ikea-stolmen-hook-three-pieces (Autodesk Fusion 360 design; units mm, degrees)
Autodesk Fusion 360 part; units mm, degrees
note: some values were not read from the file. Set by a fixed rule: which sketch regions a step uses.
sketch "Sketch1" plane through (0, 0, 0) normal (0, 1, 0) x (1, 0, 0) in component "Component"
  circle A0 centre (0, 0) radius 23.5
  circle A1 centre (0, 0) radius 27.5
  line L0 (-5, 35.5) -> (-9, 35.5)
  line L1 (-9, 35.5) -> (-9, 23.5)
  line L2 (-9, 23.5) -> (-5, 23.5)
  line L3 (-5, 23.5) -> (-5, 35.5)
  line L4 (0, 5) -> (0, -5)
  line L5 (-5, 0) -> (5, 0)
  line L6 (9, 35.5) -> (9, 23.5)
  line L7 (5, 23.5) -> (5, 35.5)
  line L8 (9, 23.5) -> (5, 23.5)
  line L9 (5, 35.5) -> (9, 35.5)
  line L10 (-9, -35.5) -> (-9, -23.5)
  line L11 (-5, -23.5) -> (-5, -35.5)
  line L12 (5, -23.5) -> (5, -35.5)
  line L13 (9, -35.5) -> (9, -23.5)
  line L14 (5, -35.5) -> (9, -35.5)
  line L15 (9, -23.5) -> (5, -23.5)
  line L16 (-9, -23.5) -> (-5, -23.5)
  line L17 (-5, -35.5) -> (-9, -35.5)
  line L18 (-5, 23.5) -> (-5, -23.5)
  line L19 (5, -23.5) -> (5, 23.5)
  dimension "d2" = 47
  dimension "d4" = 55
  dimension "d7" = 4
  dimension "d54" = 12
  measures "d2" diameter of A0
  measures "d4" diameter of A1
  measures "d7" distance of L0.start L0.end
  measures "d54" distance of L0.end L1.end
extrude "Extrude1" add sketch "Sketch1" along normal blind 10 contours A0 A1 L6 L8 L13 L15 L19 | A1 L6 L7 L8 | A1 L12 L13 L15 | A1 L6 L7 L9 | A1 L12 L13 L14 makes body 1 in component "Component"
sketch "Sketch6" plane through (9, 0, 0) normal (1, 0, 0) x (0, 0, -1)
  line L0 (-35.5, 0) -> (-25.9856, 0)
  line L1 (-25.9856, 0) -> (-25.9856, 10)
  line L2 (-25.9856, 10) -> (-35.5, 10)
  line L3 (-35.5, 10) -> (-35.5, 0)
  line L4 (-35.5, 5) -> (-25.9856, 5)
  circle A0 centre (-30.7428, 5) radius 1.6
  line L5 (-30.7428, 8.2) -> (-33.5141, 6.6)
  line L6 (-33.5141, 6.6) -> (-33.5141, 3.4)
  line L7 (-33.5141, 3.4) -> (-30.7428, 1.8)
  line L8 (-30.7428, 1.8) -> (-27.9715, 3.4)
  line L9 (-27.9715, 3.4) -> (-27.9715, 6.6)
  line L10 (-27.9715, 6.6) -> (-30.7428, 8.2)
  line L11 (-30.7428, 7.4) -> (-31.9354, 6.0667)
  line L12 (-30.7428, 7.4) -> (-29.5502, 6.0667)
  point P0 (-30.7428, 5)
  dimension "d72" = 3.2
  dimension "d78" = 2.4
  measures "d72" diameter of A0
  measures "d78" distance of P0 L11.start
sketch "Sketch7" plane through (9, 0, 0) normal (1, 0, 0) x (0, 0, -1)
  line L0 (25.9856, 0) -> (35.5, 0)
  line L1 (35.5, 0) -> (35.5, 10)
  line L2 (35.5, 10) -> (25.9856, 10)
  line L3 (25.9856, 10) -> (25.9856, 0)
  line L4 (25.9856, 5) -> (35.5, 5)
  circle A0 centre (30.7428, 5) radius 1.6
  line L5 (30.7428, 5) -> (30.7428, 7.4)
  line L6 (30.7428, 7.4) -> (29.5502, 6.0667)
  line L7 (30.7428, 7.4) -> (31.9354, 6.0667)
  dimension "d73" = 3.2
  dimension "d79" = 2.4
  measures "d73" diameter of A0
  measures "d79" distance of A0.centre L5.end
extrude "Extrude5" cut sketch "Sketch6" against normal up to surface (4 mm away) contours L4 A0 | L4 A0 | A0 L11 L12 bodies 1 in component "Component"
extrude "Extrude6" cut sketch "Sketch7" against normal up to surface (4 mm away) contours L4 A0 L5 | L4 A0 | L4 A0 L5 | A0 L5 L6 | A0 L5 L7 bodies 1 in component "Component"
extrude "Extrude7" cut sketch "Sketch6" against normal blind 1.5 contours L4 A0 L5 L6 L9 L10 L11 L12 | L4 A0 L6 L7 L8 L9 | A0 L11 L12 bodies 1 in component "Component"
sketch "Sketch5" plane through (0, 0, 0) normal (0, 1, 0) x (1, 0, 0)
  circle A0 centre (-14.9966, 15) radius 5
  line L0 (-19.9966, 15) -> (-19.9966, 0)
  line L1 (-9.9966, 15) -> (-9.9966, 0)
  circle A1 centre (-14.9966, 15) radius 1.6
  line L2 (-14.9966, 2) -> (-6.4966, 2)
  line L3 (-6.4966, 2) -> (-6.4966, -2)
  line L4 (-6.4966, -2) -> (-14.9966, -2)
  line L5 (-14.9966, -2) -> (-14.9966, 2)
  line L6 (-19.9966, 0) -> (-9.9966, 0)
  arc A2 (-49.9966, 0) -> (-19.9966, 0) centre (-34.9966, 0) ccw
  line L7 (-34.9966, 0) -> (-49.9966, 0) construction
  line L8 (-34.9966, 0) -> (-19.9966, 0) construction
  arc A3 (-59.9966, 0) -> (-9.9966, 0) centre (-34.9966, 0) ccw
  line L9 (-34.9966, 0) -> (-59.9966, 0) construction
  line L10 (-34.9966, 0) -> (-9.9966, 0) construction
  line L11 (-49.9966, 0) -> (-59.9966, 0)
  arc A4 (-49.9966, 0) -> (-59.9966, 0) centre (-54.9966, 0) ccw
  dimension "d64" = 10
  dimension "d65" = 8
  dimension "d67" = 3.2
  dimension "d68" = 8.5
  dimension "d74" = 180
  dimension "d75" = 15
  dimension "d76" = 180
  measures "d64" diameter of A0
  measures "d67" diameter of A1
  measures "d68" distance of L3.end L4.end
  measures "d74" angle of L7 L8
  measures "d75" distance of L0.end A2.centre
  measures "d76" angle of L9 L10
extrude "Extrude2" add sketch "Sketch5" along normal blind 8.5 separate body makes body 2
fillet "Fillet5" radius 3 2 edges at (-10.0767, 4.25, 2) (-9.9966, 4.25, -2) on bodies 2
component "Component" placed x (1, 0, 0) y (0, 1, 0) z (0, 0, 1) at (0, 0, 0)
equation "ikeaStolmanPoleDiameter = 47 mm"
equation "d2 = ikeaStolmanPoleDiameter"
equation "thickness = 4 mm"
equation "d4 = ikeaStolmanPoleDiameter + thickness + thickness"
equation "d7 = thickness"
equation "d11 = height"
equation "flexThickness = 0.75 mm"
equation "height = 10 mm"
equation "d64 = height"
